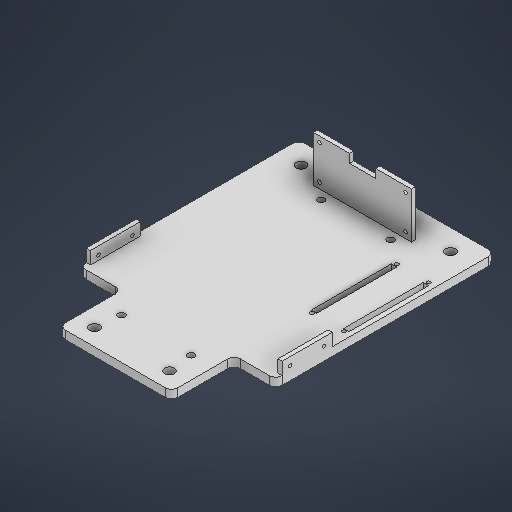
# Autodesk Inventor part: 1.5_base
Saved by Autodesk Inventor 2025 (Build 290162010, 162A)
## iProperties
Created: 2024-05-22
Part Number: 1.5_base
Material: Generic
Document SubType Name: Modeling
Designer: Garfieldcmix
Density: 1 g/cm^3
Appearance: Default
Author: Garfieldcmix
Autodesk Inventor part; units mm, degrees
ref_plane "YZ Plane" through (0, 0, 0) normal (1, 0, 0) x (0, 1, 0)
ref_plane "XZ Plane" through (0, 0, 0) normal (0, 1, 0) x (-1, 0, 0)
ref_plane "XY Plane" through (0, 0, 0) normal (0, 0, 1) x (1, 0, 0)
derived "Car_Plan.ipt"
sketch "Car_Sketch" plane through (0, 0, 0) normal (0, 1, 0) x (-1, 0, 0)
  line L0 (0, 0) -> (94, 0)
  line L1 (0, 0) -> (0, 105)
  line L2 (94, 0) -> (94, 105)
  line L3 (0, 105) -> (20, 105)
  line L4 (20, 105) -> (20, 190)
  line L5 (20, 190) -> (74, 190)
  line L6 (74, 190) -> (74, 105)
  line L7 (74, 105) -> (94, 105)
  line L8 (-5, 68) -> (-5, 0)
  line L9 (-5, 0) -> (-32, 0)
  line L10 (-32, 0) -> (-32, 68)
  line L11 (-32, 68) -> (-5, 68)
  line L12 (47, 190) -> (47, 0) construction
  line L13 (126, 68) -> (99, 68)
  line L14 (99, 68) -> (99, 0)
  line L15 (126, 0) -> (126, 68)
  line L16 (99, 0) -> (126, 0)
  line L17 (-5, 34) -> (99, 34) construction
  line L18 (0, 95) -> (94, 95) construction
  line L19 (-5, 190) -> (-32, 190)
  line L20 (-32, 122) -> (-5, 122)
  line L21 (-32, 190) -> (-32, 122)
  line L22 (-5, 122) -> (-5, 190)
  line L23 (-5, 156) -> (99, 156) construction
  line L24 (126, 122) -> (99, 122)
  line L25 (126, 190) -> (126, 122)
  line L26 (99, 190) -> (126, 190)
  line L27 (99, 122) -> (99, 190)
  line L28 (0, 156) -> (47, 34) construction
  line L29 (94, 156) -> (47, 34) construction
  line L30 (0, 156) -> (-174.2341, 34) construction
  line L31 (-5, 34) -> (-174.2341, 34) construction
  line L32 (8.9873, 132.6713) -> (47, 141.55) construction
  line L33 (85.0127, 132.6713) -> (47, 141.55) construction
sketch "Base" plane through (0, 0, 0) normal (0, 1, 0) x (-1, 0, 0)
  line L0 (0, 0) -> (0, 105) projected
  line L1 (0, 105) -> (20, 105) projected
  line L2 (20, 105) -> (20, 190) projected
  line L3 (74, 190) -> (74, 105) projected
  line L4 (74, 105) -> (94, 105) projected
  line L5 (94, 0) -> (94, 105) projected
  line L6 (0, 0) -> (94, 0) projected
  line L7 (74, 135) -> (20, 135)
  circle A0 centre (29, 127) radius 2.4
  circle A1 centre (65, 127) radius 2.4
  circle A2 centre (11.1, 10) radius 2.4
  circle A3 centre (82.9, 10) radius 2.4
  dimension "d76" = 30
  dimension "d77" = 4.8
  dimension "d78" = 4.8
  dimension "d79" = 9
  dimension "d80" = 22
  dimension "d81" = 22
  dimension "d82" = 9
  dimension "d83" = 4.8
  dimension "d84" = 4.8
  dimension "d85" = 10
  dimension "d86" = 11.1
  dimension "d87" = 10
  dimension "d88" = 11.1
  constraints: 4 centre point, 2 end point, 2 point on line, 1 perpendicular
  measures "d76" distance between parallel lines of L1 L7
  measures "d77" diameter of A0
  measures "d78" diameter of A1
  measures "d79" distance from line of L2 A0.centre
  measures "d80" distance from line of L1 A0.centre
  measures "d81" distance from line of A1.centre L4
  measures "d82" distance from line of L3 A1.centre
  measures "d83" diameter of A2
  measures "d84" diameter of A3
  measures "d85" distance from line of L6 A2.centre
  measures "d86" distance from line of L0 A2.centre
  measures "d87" distance from line of L6 A3.centre
  measures "d88" distance from line of L5 A3.centre
extrude "Extrusion1" add sketch "Base" along normal blind 4
fillet "Fillet2" radius 3 8 edges at (-20, 2, 105) (0, 2, 105) (0, 2, 0) (-94, 2, 0) (-94, 2, 105) (-74, 2, 105) (-74, 2, 135) (-20, 2, 135)
sketch "Sketch9" plane through (0, 4, 0) normal (0, 1, 0) x (1, 0, 0)
  line L0 (0, -102) -> (0, -3) projected
  line L1 (0, -101.967) -> (-2, -101.967)
  line L2 (-2, -101.967) -> (-2, -77.967)
  line L3 (-2, -77.967) -> (0, -77.967)
  line L4 (0, -77.967) -> (0, -101.967)
  line L5 (-71, -135) -> (-23, -135) projected
  line L6 (-47, -135) -> (-47, -94.1644)
  line L7 (0, -102) -> (0, -3) projected
  line L8 (-17, -105) -> (-3, -105) projected
  line L9 (0, -102) -> (0, -77.967)
  line L10 (-94, -101.967) -> (-92, -101.967)
  line L11 (-92, -101.967) -> (-92, -77.967)
  line L12 (-92, -77.967) -> (-94, -77.967)
  line L13 (-94, -3) -> (-94, -102) projected
  line L14 (-94, -102) -> (-94, -77.967)
  point P0 (0, 0)
  point P1 (0, -77.967)
  dimension "d105" = 2
  dimension "d106" = 24
  dimension "d107" = 3.033
  constraints: 20 end point, 4 symmetric about line, 3 perpendicular, 2 parallel, 1 collinear, 1 horizontal, 1 midpoint, 1 point on line, 1 vertical
  measures "d105" distance of L2.end L3.end
  measures "d106" distance of L1.end L2.end
  measures "d107" distance between parallel lines of L8 L1
extrude "left-ultrasonic-holder" add sketch "Sketch9" along normal blind 6
sketch "Sketch10" plane through (0, 0, 102) normal (1, 0, 0) x (0, 0, -1)
  line L0 (0.033, 10) -> (24.033, 10) projected
  line L1 (0.033, 10) -> (3.833, 10)
  line L2 (0.033, 6.2) -> (0.033, 10)
  circle A0 centre (3.833, 6.2) radius 0.85
  line L3 (0.033, 4) -> (0.033, 10) projected
  circle A1 centre (20.133, 6.2) radius 0.85
  line L4 (24.033, 4) -> (24.033, 10) projected
  point P0 (102, 0)
  dimension "d112" = 1.7
  dimension "d113" = 3.8
  dimension "d114" = 3.8
  dimension "d125" = 16.3
  dimension "d126" = 3.9
  dimension "d127" = 3.8
  dimension "d128" = 1.7
  dimension "d190" = 90
  constraints: 4 end point, 2 centre point, 1 horizontal
  measures "d112" diameter of A0
  measures "d113" distance from line of L3 A0.centre
  measures "d114" distance from line of L0 A0.centre
  measures "d125" distance of A1.centre A0.centre
  measures "d126" distance from line of L4 A1.centre
  measures "d127" distance from line of L0 A1.centre
  measures "d128" diameter of A1
  measures "d190" angle of L0 L2
extrude "holder-hole1" cut sketch "Sketch10" against normal blind 2
sketch "Sketch11" plane through (-94, 0, 3) normal (-1, 0, 0) x (0, 0, 1)
  line L0 (74.967, 4) -> (74.967, 10) projected
  line L1 (74.967, 10) -> (78.767, 10)
  line L2 (74.967, 6.2) -> (74.967, 10)
  circle A0 centre (78.767, 6.2) radius 0.85
  line L3 (74.967, 10) -> (98.967, 10) projected
  circle A1 centre (95.067, 6.2) radius 0.85
  line L4 (98.967, 4) -> (98.967, 10) projected
  point P0 (-3, 0)
  dimension "d119" = 1.7
  dimension "d120" = 3.8
  dimension "d121" = 3.8
  dimension "d129" = 16.3
  dimension "d130" = 3.9
  dimension "d131" = 1.7
  constraints: 4 end point, 2 centre point, 1 horizontal
  measures "d119" diameter of A0
  measures "d120" distance from line of L3 A0.centre
  measures "d121" distance from line of L0 A0.centre
  measures "d129" distance of A1.centre A0.centre
  measures "d130" distance from line of L4 A1.centre
  measures "d131" diameter of A1
extrude "holder-hole2" cut sketch "Sketch11" against normal blind 2
sketch "Sketch12" plane through (0, 4, 0) normal (0, 1, 0) x (1, 0, 0)
  line L0 (-3, 0) -> (-91, 0) projected
  line L1 (-47, 0) -> (-24.5, 0)
  line L2 (-24.5, 0) -> (-24.5, -13.4)
  line L3 (-24.5, -13.4) -> (-71.5, -13.4)
  line L4 (-71.5, -13.4) -> (-71.5, -15.4)
  line L5 (-71.5, -15.4) -> (-24.5, -15.4)
  line L6 (-24.5, -15.4) -> (-24.5, -13.4)
  point P0 (0, 0)
  dimension "d132" = 22.5
  dimension "d134" = 13.4
  dimension "d135" = 47
  dimension "d136" = 2
  constraints: 12 end point, 2 parallel, 1 horizontal, 1 midpoint, 1 perpendicular, 1 point on line, 1 vertical
  measures "d132" distance of L1.start L1.end
  measures "d134" distance of L1.end L2.end
  measures "d135" distance of L5.end L4.end
  measures "d136" distance of L4.end L3.end
extrude "back-ultrasonic-holder" add sketch "Sketch12" along normal blind 22
sketch "Sketch13" plane through (-24.5, 4, 13.4) normal (0, 0, -1) x (-1, 0, 0)
  line L0 (47, 22) -> (0, 22) projected
  line L1 (0, 22) -> (2.85, 22)
  line L2 (0, 19.15) -> (0, 22)
  circle A0 centre (2.85, 19.15) radius 0.85
  line L3 (0, 0) -> (0, 22) projected
  circle A1 centre (44.15, 19.15) radius 0.85
  line L4 (0, 11) -> (20.2674, 11)
  circle A2 centre (2.85, 2.85) radius 0.85
  circle A3 centre (44.15, 2.85) radius 0.85
  line L5 (23.5, 22) -> (17.25, 22)
  line L6 (17.25, 22) -> (29.75, 22)
  line L7 (29.75, 22) -> (29.75, 17.8348)
  line L8 (29.75, 17.8348) -> (17.25, 17.8348)
  line L9 (17.25, 17.8348) -> (17.25, 22)
  line L10 (47, 0) -> (47, 22) projected
  point P0 (-24.5, -4)
  point P1 (1.425, 22)
  point P2 (29.75, 22)
  dimension "d141" = 1.7
  dimension "d142" = 2.85
  dimension "d143" = 2.85
  dimension "d146" = 6.25
  dimension "d147" = 12.5
  dimension "d148" = 2.85
  dimension "d149" = 2.85
  dimension "d150" = 1.7
  dimension "d185" = 20.2674
  constraints: 16 end point, 4 centre point, 3 horizontal, 3 midpoint, 2 parallel, 2 symmetric about line, 1 perpendicular, 1 point on line, 2 other
  measures "d141" diameter of A0
  measures "d142" distance from line of L3 A0.centre
  measures "d143" vertical distance of point (1.425, 22) A0.centre
  measures "d146" distance of L5.start L5.end
  measures "d147" distance of L7.end L8.end
  measures "d148" distance from line of L10 A1.centre
  measures "d149" distance from line of L0 A1.centre
  measures "d150" diameter of A1
  measures "d185" distance of L4.start L4.end
extrude "back-holder-hole" cut sketch "Sketch13" against normal blind 2
sketch "Sketch14" plane through (0, 4, 0) normal (0, 1, 0) x (1, 0, 0)
  line L0 (0, -102) -> (0, -3) projected
  line L1 (0, -70) -> (-2.25, -70)
  line L2 (0, -77.967) -> (0, -3) projected
  line L3 (-3, 0) -> (-91, 0) projected
  line L4 (-2.25, -70) -> (-20.25, -70)
  line L5 (-20.25, -70) -> (-20.25, -26.8)
  line L6 (-20.25, -26.8) -> (-2.25, -26.8)
  line L7 (-2.25, -26.8) -> (-2.25, -70)
  line L8 (-2.25, -70) -> (-3.63, -70)
  line L9 (-2.25, -68.72) -> (-2.25, -70)
  circle A0 centre (-3.63, -68.72) radius 0.9
  line L10 (-11.25, -70) -> (-11.25, -64.8445)
  circle A1 centre (-18.87, -68.72) radius 0.9
  line L11 (-2.25, -48.4) -> (-9.2486, -48.4)
  circle A2 centre (-3.63, -28.08) radius 0.9
  circle A3 centre (-18.87, -28.08) radius 0.9
  line L12 (-2.25, -67.5978) -> (-4.85, -67.5978)
  line L13 (-4.85, -67.5978) -> (-4.85, -29.313)
  line L14 (-4.85, -29.313) -> (-2.25, -29.313)
  line L15 (-2.25, -29.313) -> (-2.25, -67.5978)
  line L16 (-20.25, -67.5978) -> (-17.65, -67.5978)
  line L17 (-17.65, -67.5978) -> (-17.65, -29.313)
  line L18 (-17.65, -29.313) -> (-20.25, -29.313)
  point P0 (0, 0)
  dimension "d151" = 2.25
  dimension "d152" = 70
  dimension "d153" = 18
  dimension "d154" = 43.2
  dimension "d157" = 1.8
  dimension "d158" = 1.28
  dimension "d159" = 1.38
  dimension "d162" = 2.6
  dimension "d186" = 2.4022
  dimension "d187" = 2.513
  constraints: 32 end point, 7 symmetric about line, 5 horizontal, 4 centre point, 4 parallel, 3 perpendicular, 2 midpoint, 2 point on line, 1 vertical, 3 other
  measures "d151" distance of L1.start L1.end
  measures "d152" distance between parallel lines of L3 L1
  measures "d153" distance of L5.end L6.end
  measures "d154" distance of L4.end L5.end
  measures "d157" diameter of A0
  measures "d158" distance from line of L4 A0.centre
  measures "d159" distance from line of L7 A0.centre
  measures "d162" distance of L13.end L14.end
  measures "d186" distance between parallel lines of L4 L12
  measures "d187" distance between parallel lines of L6 L18
extrude "arduino-hole" cut sketch "Sketch14" against normal through all contours L12 L13 L11 L7 | L11 L13 L14 L7 | L5 L18 L17 L16 | A0 | A1 | A2 | A3
sketch "Sketch15" plane through (0, 4, 0) normal (0, 1, 0) x (1, 0, 0)
  line L0 (0, -101.967) -> (0, -77.967) projected
  line L1 (0, -94.8628) -> (-2.5, -94.8628)
  circle A0 centre (-4.75, -92.6128) radius 1.5
  line L2 (-4.75, -84.6128) -> (-10.6955, -84.6128)
  circle A1 centre (-4.75, -76.6128) radius 1.5
  line L3 (-17, -105) -> (-3, -105) projected
  line L4 (0, -77.967) -> (0, -3) projected
  point P0 (0, 0)
  dimension "d166" = 3
  dimension "d167" = 8
  dimension "d168" = 4.75
  dimension "d169" = 12.3872
  dimension "d170" = 4.75
  dimension "d171" = 28.3872
  dimension "d188" = 2.5
  dimension "d189" = 2.25
  constraints: 4 end point, 2 centre point, 1 horizontal, 1 point on line, 1 symmetric about line, 1 other
  measures "d166" diameter of A0
  measures "d167" distance of A0.centre L2.start
  measures "d168" distance from line of L0 A0.centre
  measures "d169" distance from line of L3 A0.centre
  measures "d170" distance from line of L4 A1.centre
  measures "d171" distance from line of L3 A1.centre
  measures "d188" distance of L1.start L1.end
  measures "d189" distance from line of A0.centre L1
extrude "MPU-hole" cut sketch "Sketch15" against normal through all
sketch "Sketch17" plane through (0, 4, 0) normal (0, 1, 0) x (1, 0, 0)
  line L0 (-20, -132) -> (-20, -108) projected
  line L1 (-20, -117.5) -> (-23.7, -117.5)
  line L2 (-20, -132) -> (-20, -108) projected
  line L3 (-71, -135) -> (-23, -135) projected
  line L4 (-23.7, -117.5) -> (-70.3, -117.5)
  line L5 (-70.3, -117.5) -> (-70.3, -17.4)
  line L6 (-70.3, -17.4) -> (-23.7, -17.4)
  line L7 (-23.7, -17.4) -> (-23.7, -117.5)
  line L8 (-23.7, -117.5) -> (-30.35, -117.5)
  line L9 (-23.7, -115.35) -> (-23.7, -117.5)
  circle A0 centre (-30.35, -115.35) radius 1.65
  line L10 (-47, -117.5) -> (-47, -109.6456)
  line L11 (-23.7, -67.45) -> (-42.2695, -67.45)
  circle A1 centre (-63.65, -115.35) radius 1.65
  line L12 (-70.3, -67.45) -> (-51.7305, -67.45)
  circle A2 centre (-30.35, -19.55) radius 1.65
  circle A3 centre (-63.65, -19.55) radius 1.65
  point P0 (0, 0)
  dimension "d174" = 3.7
  dimension "d175" = 17.5
  dimension "d176" = 46.6
  dimension "d177" = 100.1
  dimension "d180" = 3.3
  dimension "d181" = 2.15
  dimension "d182" = 6.65
  constraints: 20 end point, 5 symmetric about line, 4 centre point, 4 horizontal, 2 midpoint, 2 parallel, 2 perpendicular, 1 point on line, 1 vertical, 3 other
  measures "d174" distance of L1.start L1.end
  measures "d175" distance between parallel lines of L3 L1
  measures "d176" distance of L5.end L6.end
  measures "d177" distance of L4.end L5.end
  measures "d180" diameter of A0
  measures "d181" distance from line of L4 A0.centre
  measures "d182" distance from line of L7 A0.centre
extrude "battery-hole" cut sketch "Sketch17" against normal through all contours A0 | A1 | A2 | A3
body "Solid1"
